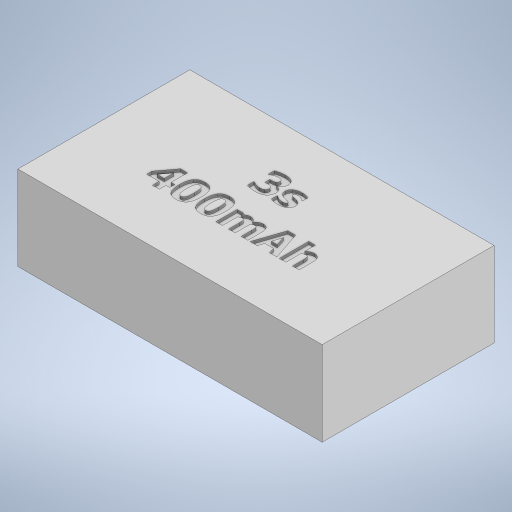
# Autodesk Inventor part: li_po3s_400mAh
Saved by Autodesk Inventor 2023 (Build 270158000, 158)
## iProperties
Created: 2025-03-19
Part Number: li_po3s_400mAh
Material: Ogólny
Document SubType Name: Modeling
Designer: kamil
Density: 1 g/cm^3
Appearance: Domyślna
Author: kamil
Autodesk Inventor part; units mm, degrees
ref_plane "YZ Plane" through (0, 0, 0) normal (1, 0, 0) x (0, 1, 0)
ref_plane "XZ Plane" through (0, 0, 0) normal (0, 1, 0) x (-1, 0, 0)
ref_plane "XY Plane" through (0, 0, 0) normal (0, 0, 1) x (1, 0, 0)
sketch "Szkic1" plane through (0, 0, 0) normal (0, 1, 0) x (-1, 0, 0)
  line L0 (4.6678, 11.8796) -> (-49.3322, 11.8796)
  line L1 (-49.3322, 11.8796) -> (-49.3322, -18.6204)
  line L2 (-49.3322, -18.6204) -> (4.6678, -18.6204)
  line L3 (4.6678, -18.6204) -> (4.6678, 11.8796)
  point P0 (0, 0)
  dimension "d0" = 54
  dimension "d1" = 30.5
  constraints: 8 end point, 2 parallel, 1 horizontal, 1 perpendicular
  measures "d0" distance of L2.end L1.end
  measures "d1" distance of L1.end L0.end
extrude "Wyciągnięcie proste1" add sketch "Szkic1" along normal blind 15
sketch "Szkic2" plane through (0, 15, 0) normal (0, 1, 0) x (1, 0, 0)
  line L0 (9.9953, 13.2196) -> (33.64, 13.2196) construction
  line L1 (33.64, 13.2196) -> (33.64, -4.8364) construction
  line L2 (33.64, -4.8364) -> (9.9953, -4.8364) construction
  line L3 (9.9953, -4.8364) -> (9.9953, 13.2196) construction
  spline S0 degree 2 poles (21.9149, 7.3232) (21.9149, 6.9544) (21.6434, 6.3507) (21.3801, 6.14) knots 0 0 0 1 2 2 2
  spline S1 degree 2 poles (21.3801, 6.14) (21.1167, 5.9293) (20.3995, 5.7024) (19.8849, 5.7024) knots 0 0 0 1 2 2 2
  spline S2 degree 2 poles (19.8849, 5.7024) (19.3015, 5.7024) (18.4668, 5.8969) (18.2034, 6.0185) knots 0 0 0 1 2 2 2
  line L4 (18.2034, 6.0185) -> (18.2034, 7.1044)
  line L5 (18.2034, 7.1044) -> (18.325, 7.1044)
  spline S3 degree 2 poles (18.325, 7.1044) (18.6005, 6.9301) (19.342, 6.6708) (19.6499, 6.6708) knots 0 0 0 1 2 2 2
  spline S4 degree 2 poles (19.6499, 6.6708) (19.8323, 6.6708) (20.2577, 6.7356) (20.4036, 6.841) knots 0 0 0 1 2 2 2
  spline S5 degree 2 poles (20.4036, 6.841) (20.517, 6.9261) (20.6548, 7.1732) (20.6548, 7.3961) knots 0 0 0 1 2 2 2
  spline S6 degree 2 poles (20.6548, 7.3961) (20.6548, 7.6189) (20.4603, 7.858) (20.2982, 7.9147) knots 0 0 0 1 2 2 2
  spline S7 degree 2 poles (20.2982, 7.9147) (20.1361, 7.9715) (19.6864, 7.9836) (19.5122, 7.9836) knots 0 0 0 1 2 2 2
  line L6 (19.5122, 7.9836) -> (19.2974, 7.9836)
  line L7 (19.2974, 7.9836) -> (19.2974, 8.8629)
  line L8 (19.2974, 8.8629) -> (19.4959, 8.8629)
  spline S8 degree 2 poles (19.4959, 8.8629) (19.7229, 8.8629) (20.1078, 8.9034) (20.2415, 8.9642) knots 0 0 0 1 2 2 2
  spline S9 degree 2 poles (20.2415, 8.9642) (20.3752, 9.029) (20.5251, 9.2559) (20.5251, 9.4504) knots 0 0 0 1 2 2 2
  spline S10 degree 2 poles (20.5251, 9.4504) (20.5251, 9.6044) (20.3833, 9.7948) (20.282, 9.8475) knots 0 0 0 1 2 2 2
  spline S11 degree 2 poles (20.282, 9.8475) (20.1605, 9.9082) (19.8363, 9.9488) (19.7229, 9.9488) knots 0 0 0 1 2 2 2
  spline S12 degree 2 poles (19.7229, 9.9488) (19.5405, 9.9488) (19.1556, 9.8637) (18.9773, 9.7948) knots 0 0 0 1 2 2 2
  spline S13 degree 2 poles (18.9773, 9.7948) (18.8355, 9.7421) (18.5276, 9.5719) (18.4546, 9.5274) knots 0 0 0 1 2 2 2
  line L9 (18.4546, 9.5274) -> (18.3493, 9.5274)
  line L10 (18.3493, 9.5274) -> (18.3493, 10.5971)
  spline S14 degree 2 poles (18.3493, 10.5971) (18.6086, 10.7065) (19.4838, 10.9131) (19.9417, 10.9131) knots 0 0 0 1 2 2 2
  spline S15 degree 2 poles (19.9417, 10.9131) (20.3874, 10.9131) (21.0438, 10.7591) (21.2747, 10.6092) knots 0 0 0 1 2 2 2
  spline S16 degree 2 poles (21.2747, 10.6092) (21.53, 10.4512) (21.7853, 9.965) (21.7853, 9.6611) knots 0 0 0 1 2 2 2
  spline S17 degree 2 poles (21.7853, 9.6611) (21.7853, 9.2316) (21.2909, 8.5914) (20.8857, 8.4982) knots 0 0 0 1 2 2 2
  line L11 (20.8857, 8.4982) -> (20.8857, 8.4496)
  spline S18 degree 2 poles (20.8857, 8.4496) (21.064, 8.4253) (21.4044, 8.2956) (21.5665, 8.1497) knots 0 0 0 1 2 2 2
  spline S19 degree 2 poles (21.5665, 8.1497) (21.7164, 8.0201) (21.9149, 7.6068) (21.9149, 7.3232) knots 0 0 0 1 2 2 2
  spline S20 degree 2 poles (23.8355, 5.7065) (23.4222, 5.7065) (22.6807, 5.8888) (22.4376, 6.0103) knots 0 0 0 1 2 2 2
  line L12 (22.4376, 6.0103) -> (22.4376, 7.0031)
  line L13 (22.4376, 7.0031) -> (22.5348, 7.0031)
  spline S21 degree 2 poles (22.5348, 7.0031) (22.6199, 6.9382) (22.8347, 6.7843) (23.0251, 6.6992) knots 0 0 0 1 2 2 2
  spline S22 degree 2 poles (23.0251, 6.6992) (23.1912, 6.6222) (23.6005, 6.5128) (23.8436, 6.5128) knots 0 0 0 1 2 2 2
  spline S23 degree 2 poles (23.8436, 6.5128) (24.0908, 6.5128) (24.4716, 6.6668) (24.4716, 6.8329) knots 0 0 0 1 2 2 2
  spline S24 degree 2 poles (24.4716, 6.8329) (24.4716, 6.9625) (24.2974, 7.1003) (24.0462, 7.157) knots 0 0 0 1 2 2 2
  spline S25 degree 2 poles (24.0462, 7.157) (23.9125, 7.1935) (23.5032, 7.2705) (23.3452, 7.3191) knots 0 0 0 1 2 2 2
  spline S26 degree 2 poles (23.3452, 7.3191) (22.8995, 7.4569) (22.4538, 7.9958) (22.4538, 8.4374) knots 0 0 0 1 2 2 2
  spline S27 degree 2 poles (22.4538, 8.4374) (22.4538, 8.6886) (22.6848, 9.1343) (22.9117, 9.3086) knots 0 0 0 1 2 2 2
  spline S28 degree 2 poles (22.9117, 9.3086) (23.1345, 9.4787) (23.795, 9.6813) (24.2123, 9.6813) knots 0 0 0 1 2 2 2
  spline S29 degree 2 poles (24.2123, 9.6813) (24.6094, 9.6813) (25.2739, 9.5233) (25.5008, 9.4139) knots 0 0 0 1 2 2 2
  line L14 (25.5008, 9.4139) -> (25.5008, 8.4577)
  line L15 (25.5008, 8.4577) -> (25.4076, 8.4577)
  spline S30 degree 2 poles (25.4076, 8.4577) (25.3468, 8.5063) (25.0835, 8.6643) (24.9619, 8.721) knots 0 0 0 1 2 2 2
  spline S31 degree 2 poles (24.9619, 8.721) (24.812, 8.7859) (24.4473, 8.875) (24.2569, 8.875) knots 0 0 0 1 2 2 2
  spline S32 degree 2 poles (24.2569, 8.875) (24.0016, 8.875) (23.6491, 8.7008) (23.6491, 8.559) knots 0 0 0 1 2 2 2
  spline S33 degree 2 poles (23.6491, 8.559) (23.6491, 8.4293) (23.8233, 8.2834) (24.1151, 8.2105) knots 0 0 0 1 2 2 2
  spline S34 degree 2 poles (24.1151, 8.2105) (24.265, 8.174) (24.658, 8.1052) (24.8404, 8.0444) knots 0 0 0 1 2 2 2
  spline S35 degree 2 poles (24.8404, 8.0444) (25.2455, 7.9147) (25.6669, 7.4082) (25.6669, 6.9868) knots 0 0 0 1 2 2 2
  spline S36 degree 2 poles (25.6669, 6.9868) (25.6669, 6.7235) (25.4198, 6.2413) (25.1888, 6.0792) knots 0 0 0 1 2 2 2
  spline S37 degree 2 poles (25.1888, 6.0792) (24.9498, 5.9009) (24.2934, 5.7065) (23.8355, 5.7065) knots 0 0 0 1 2 2 2
  line L16 (11.6576, -1.2577) -> (10.981, -1.2577)
  line L17 (10.981, -1.2577) -> (10.981, -2.4368)
  line L18 (10.981, -2.4368) -> (9.7694, -2.4368)
  line L19 (9.7694, -2.4368) -> (9.7694, -1.2577)
  line L20 (9.7694, -1.2577) -> (7.5652, -1.2577)
  line L21 (7.5652, -1.2577) -> (7.5652, -0.3257)
  line L22 (7.5652, -0.3257) -> (9.7289, 2.5754)
  line L23 (9.7289, 2.5754) -> (10.981, 2.5754)
  line L24 (10.981, 2.5754) -> (10.981, -0.3582)
  line L25 (10.981, -0.3582) -> (11.6576, -0.3582)
  line L26 (11.6576, -0.3582) -> (11.6576, -1.2577)
  line L27 (9.7694, -0.3582) -> (9.7694, 1.3436)
  line L28 (9.7694, 1.3436) -> (8.5012, -0.3582)
  line L29 (8.5012, -0.3582) -> (9.7694, -0.3582)
  spline S38 degree 2 poles (15.9121, 0.0754) (15.9121, -0.5729) (15.7054, -1.5454) (15.4745, -1.8736) knots 0 0 0 1 2 2 2
  spline S39 degree 2 poles (15.4745, -1.8736) (15.2476, -2.1977) (14.5142, -2.53) (13.9874, -2.53) knots 0 0 0 1 2 2 2
  spline S40 degree 2 poles (13.9874, -2.53) (13.4566, -2.53) (12.7273, -2.1977) (12.4964, -1.8655) knots 0 0 0 1 2 2 2
  spline S41 degree 2 poles (12.4964, -1.8655) (12.2654, -1.5373) (12.0588, -0.5729) (12.0588, 0.0754) knots 0 0 0 1 2 2 2
  spline S42 degree 2 poles (12.0588, 0.0754) (12.0588, 0.7399) (12.2654, 1.6799) (12.5004, 2.0203) knots 0 0 0 1 2 2 2
  spline S43 degree 2 poles (12.5004, 2.0203) (12.7354, 2.3525) (13.4769, 2.6767) (13.9874, 2.6767) knots 0 0 0 1 2 2 2
  spline S44 degree 2 poles (13.9874, 2.6767) (14.5263, 2.6767) (15.2476, 2.3363) (15.4785, 2) knots 0 0 0 1 2 2 2
  spline S45 degree 2 poles (15.4785, 2) (15.7054, 1.6718) (15.9121, 0.7034) (15.9121, 0.0754) knots 0 0 0 1 2 2 2
  spline S46 degree 2 poles (14.6519, 0.0754) (14.6519, 1.0033) (14.3481, 1.7529) (13.9874, 1.7529) knots 0 0 0 1 2 2 2
  spline S47 degree 2 poles (13.9874, 1.7529) (13.6268, 1.7529) (13.3189, 1.0033) (13.3189, 0.0713) knots 0 0 0 1 2 2 2
  spline S48 degree 2 poles (13.3189, 0.0713) (13.3189, -0.8444) (13.6268, -1.6061) (13.9874, -1.6061) knots 0 0 0 1 2 2 2
  spline S49 degree 2 poles (13.9874, -1.6061) (14.344, -1.6061) (14.6519, -0.8444) (14.6519, 0.0754) knots 0 0 0 1 2 2 2
  spline S50 degree 2 poles (20.2921, 0.0754) (20.2921, -0.5729) (20.0855, -1.5454) (19.8545, -1.8736) knots 0 0 0 1 2 2 2
  spline S51 degree 2 poles (19.8545, -1.8736) (19.6276, -2.1977) (18.8942, -2.53) (18.3675, -2.53) knots 0 0 0 1 2 2 2
  spline S52 degree 2 poles (18.3675, -2.53) (17.8367, -2.53) (17.1074, -2.1977) (16.8764, -1.8655) knots 0 0 0 1 2 2 2
  spline S53 degree 2 poles (16.8764, -1.8655) (16.6455, -1.5373) (16.4388, -0.5729) (16.4388, 0.0754) knots 0 0 0 1 2 2 2
  spline S54 degree 2 poles (16.4388, 0.0754) (16.4388, 0.7399) (16.6455, 1.6799) (16.8805, 2.0203) knots 0 0 0 1 2 2 2
  spline S55 degree 2 poles (16.8805, 2.0203) (17.1155, 2.3525) (17.857, 2.6767) (18.3675, 2.6767) knots 0 0 0 1 2 2 2
  spline S56 degree 2 poles (18.3675, 2.6767) (18.9064, 2.6767) (19.6276, 2.3363) (19.8586, 2) knots 0 0 0 1 2 2 2
  spline S57 degree 2 poles (19.8586, 2) (20.0855, 1.6718) (20.2921, 0.7034) (20.2921, 0.0754) knots 0 0 0 1 2 2 2
  spline S58 degree 2 poles (19.032, 0.0754) (19.032, 1.0033) (18.7281, 1.7529) (18.3675, 1.7529) knots 0 0 0 1 2 2 2
  spline S59 degree 2 poles (18.3675, 1.7529) (18.0069, 1.7529) (17.6989, 1.0033) (17.6989, 0.0713) knots 0 0 0 1 2 2 2
  spline S60 degree 2 poles (17.6989, 0.0713) (17.6989, -0.8444) (18.0069, -1.6061) (18.3675, -1.6061) knots 0 0 0 1 2 2 2
  spline S61 degree 2 poles (18.3675, -1.6061) (18.7241, -1.6061) (19.032, -0.8444) (19.032, 0.0754) knots 0 0 0 1 2 2 2
  line L30 (25.5069, -2.4246) -> (25.5069, -0.5405)
  spline S62 degree 2 poles (25.5069, -0.5405) (25.5069, -0.2609) (25.4866, 0.12) (25.438, 0.2415) knots 0 0 0 1 2 2 2
  spline S63 degree 2 poles (25.438, 0.2415) (25.3853, 0.3631) (25.1746, 0.4725) (24.9842, 0.4725) knots 0 0 0 1 2 2 2
  spline S64 degree 2 poles (24.9842, 0.4725) (24.8505, 0.4725) (24.5912, 0.355) (24.4372, 0.2456) knots 0 0 0 1 2 2 2
  line L31 (24.4372, 0.2456) -> (24.4372, -2.4246)
  line L32 (24.4372, -2.4246) -> (23.2541, -2.4246)
  line L33 (23.2541, -2.4246) -> (23.2541, -0.5405)
  spline S65 degree 2 poles (23.2541, -0.5405) (23.2541, -0.265) (23.2297, 0.12) (23.1811, 0.2415) knots 0 0 0 1 2 2 2
  spline S66 degree 2 poles (23.1811, 0.2415) (23.1284, 0.3631) (22.9177, 0.4725) (22.7273, 0.4725) knots 0 0 0 1 2 2 2
  spline S67 degree 2 poles (22.7273, 0.4725) (22.5855, 0.4725) (22.3059, 0.3388) (22.1763, 0.2456) knots 0 0 0 1 2 2 2
  line L34 (22.1763, 0.2456) -> (22.1763, -2.4246)
  line L35 (22.1763, -2.4246) -> (21.0012, -2.4246)
  line L36 (21.0012, -2.4246) -> (21.0012, 1.3477)
  line L37 (21.0012, 1.3477) -> (22.1763, 1.3477)
  line L38 (22.1763, 1.3477) -> (22.1763, 0.9303)
  spline S68 degree 2 poles (22.1763, 0.9303) (22.4639, 1.1734) (22.9785, 1.449) (23.2986, 1.449) knots 0 0 0 1 2 2 2
  spline S69 degree 2 poles (23.2986, 1.449) (23.643, 1.449) (24.1698, 1.1208) (24.3075, 0.7926) knots 0 0 0 1 2 2 2
  spline S70 degree 2 poles (24.3075, 0.7926) (24.6438, 1.1086) (25.2435, 1.449) (25.5515, 1.449) knots 0 0 0 1 2 2 2
  spline S71 degree 2 poles (25.5515, 1.449) (25.8148, 1.449) (26.2322, 1.2828) (26.374, 1.1127) knots 0 0 0 1 2 2 2
  spline S72 degree 2 poles (26.374, 1.1127) (26.532, 0.9303) (26.69, 0.432) (26.69, 0.0308) knots 0 0 0 1 2 2 2
  line L39 (26.69, 0.0308) -> (26.69, -2.4246)
  line L40 (26.69, -2.4246) -> (25.5069, -2.4246)
  line L41 (27.0912, -2.4246) -> (28.7808, 2.5754)
  line L42 (28.7808, 2.5754) -> (30.1503, 2.5754)
  line L43 (30.1503, 2.5754) -> (31.84, -2.4246)
  line L44 (31.84, -2.4246) -> (30.5474, -2.4246)
  line L45 (30.5474, -2.4246) -> (30.2354, -1.4035)
  line L46 (30.2354, -1.4035) -> (28.6633, -1.4035)
  line L47 (28.6633, -1.4035) -> (28.3472, -2.4246)
  line L48 (28.3472, -2.4246) -> (27.0912, -2.4246)
  line L49 (29.9599, -0.4959) -> (29.4494, 1.1572)
  line L50 (29.4494, 1.1572) -> (28.9348, -0.4959)
  line L51 (28.9348, -0.4959) -> (29.9599, -0.4959)
  line L52 (35.7986, -2.4246) -> (34.6155, -2.4246)
  line L53 (34.6155, -2.4246) -> (34.6155, -0.5567)
  spline S73 degree 2 poles (34.6155, -0.5567) (34.6155, -0.3257) (34.579, 0.1281) (34.5304, 0.2334) knots 0 0 0 1 2 2 2
  spline S74 degree 2 poles (34.5304, 0.2334) (34.4696, 0.3631) (34.2427, 0.4725) (34.0482, 0.4725) knots 0 0 0 1 2 2 2
  spline S75 degree 2 poles (34.0482, 0.4725) (33.9064, 0.4725) (33.6106, 0.3631) (33.4445, 0.2456) knots 0 0 0 1 2 2 2
  line L54 (33.4445, 0.2456) -> (33.4445, -2.4246)
  line L55 (33.4445, -2.4246) -> (32.2694, -2.4246)
  line L56 (32.2694, -2.4246) -> (32.2694, 2.7982)
  line L57 (32.2694, 2.7982) -> (33.4445, 2.7982)
  line L58 (33.4445, 2.7982) -> (33.4445, 0.9303)
  spline S76 degree 2 poles (33.4445, 0.9303) (33.7322, 1.1734) (34.2792, 1.449) (34.6114, 1.449) knots 0 0 0 1 2 2 2
  spline S77 degree 2 poles (34.6114, 1.449) (35.1868, 1.449) (35.7986, 0.7196) (35.7986, 0.0308) knots 0 0 0 1 2 2 2
  line L59 (35.7986, 0.0308) -> (35.7986, -2.4246)
  point P0 (0, 0)
  constraints: 2 other
extrude "Wyciągnięcie proste2" cut sketch "Szkic2" against normal blind 0.5
